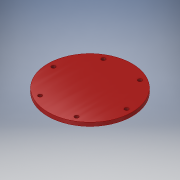
# Autodesk Inventor part: SupportPlateForWater
Saved by Autodesk Inventor 2019.1 (Build 231200000, 200)
## iProperties
Created: 2017-11-20
Part Number: SupportPlateForWater
Material: PET Plastic
Document SubType Name: Modeling
Designer: steele
Density: 1.541 g/cm^3
Appearance: Red
Author: steele
Autodesk Inventor part; units mm, degrees
ref_plane "YZ Plane" through (0, 0, 0) normal (1, 0, 0) x (0, 1, 0)
ref_plane "XZ Plane" through (0, 0, 0) normal (0, 1, 0) x (-1, 0, 0)
ref_plane "XY Plane" through (0, 0, 0) normal (0, 0, 1) x (1, 0, 0)
sketch "Sketch1" plane through (0, 0, 0) normal (0, 1, 0) x (-1, 0, 0)
  circle A0 centre (0, 0) radius 73.025
  dimension "d4" = 146.05
  constraints: 1 centre point, 1 coincident
  measures "d4" diameter of A0
extrude "Extrusion1" add sketch "Sketch1" against normal blind 6.35
sketch "Sketch7" plane through (0, 0, 0) normal (0, 1, 0) x (1, 0, 0)
  circle A0 centre (-63.5, 0) radius 3.3782
  circle A1 centre (-31.75, -54.9926) radius 3.3782
  circle A2 centre (31.75, -54.9926) radius 3.3782
  circle A3 centre (63.5, 0) radius 3.3782
  circle A4 centre (31.75, 54.9926) radius 3.3782
  circle A5 centre (-31.75, 54.9926) radius 3.3782
  point P0 (0, 0)
  dimension "d32" = 6.7564
  dimension "d33" = 63.5
  dimension "d36" = 360
  constraints: 6 centre point, 13 other
  measures "d32" diameter of A0
  measures "d33" distance of A0.centre point (0, 0)
extrude "Extrusion5" cut sketch "Sketch7" against normal through all
body "Solid1"
